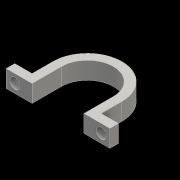
# Autodesk Inventor part: holder
Saved by Autodesk Inventor 2016 (Build 200138000, 138)
## iProperties
Created: 2019-02-07
Part Number: holder
Material: Generic
Document SubType Name: Modeling
Designer: Calb3e
Density: 1 g/cm^3
Appearance: Default
Author: Calb3e
Autodesk Inventor part; units mm, degrees
ref_plane "YZ Plane" through (0, 0, 0) normal (1, 0, 0) x (0, 1, 0)
ref_plane "XZ Plane" through (0, 0, 0) normal (0, 1, 0) x (-1, 0, 0)
ref_plane "XY Plane" through (0, 0, 0) normal (0, 0, 1) x (1, 0, 0)
sketch "Sketch1" plane through (0, 0, 0) normal (0, 0, 1) x (1, 0, 0)
  arc A0 (15, 17) -> (-15, 17) centre (0, 17) ccw
  line L0 (20, 17) -> (20, 0)
  line L1 (-20, 17) -> (-20, 0)
  line L2 (30, 5) -> (30, 0)
  line L3 (30, 0) -> (-30, 0)
  line L4 (-30, 0) -> (-30, 5)
  line L5 (15, 17) -> (15, 0)
  line L6 (-15, 17) -> (-15, 0)
  arc A1 (20, 17) -> (-20, 17) centre (0, 17) ccw
  line L7 (-30, 5) -> (-20, 5)
  line L8 (20, 5) -> (30, 5)
  point P0 (0, 0)
  point P1 (0, 0)
  dimension "d0" = 30
  dimension "d1" = 17
  dimension "d3" = 60
  dimension "d5" = 20
  dimension "d6" = 5
  dimension "d7" = 5
  constraints: 18 end point, 4 point on circle, 4 point on line, 4 tangent, 3 parallel, 3 perpendicular, 3 vertical, 2 centre point, 2 coincident, 2 horizontal, 1 midpoint, 1 vertical alignment
  measures "d0" diameter of A0
  measures "d1" distance of point (0, 0) A0.centre
  measures "d3" distance between parallel lines of L4 L2
  measures "d5" radius of A1
  measures "d6" distance between parallel lines of L3 L7
  measures "d7" distance between parallel lines of L3 L8
extrude "Extrusion1" add sketch "Sketch1" along normal blind 10 contours A0 L6 L3 L1 A1 L0 L5 | L0 L8 L2 L3 | L3 L4 L7 L1
hole "Hole1" at (25, 5, 5) direction (0, -1, 0) diameter 6 end through all
hole "Hole2" at (-25, 5, 5) direction (0, -1, 0) diameter 6 end through all
body "Solid1"
